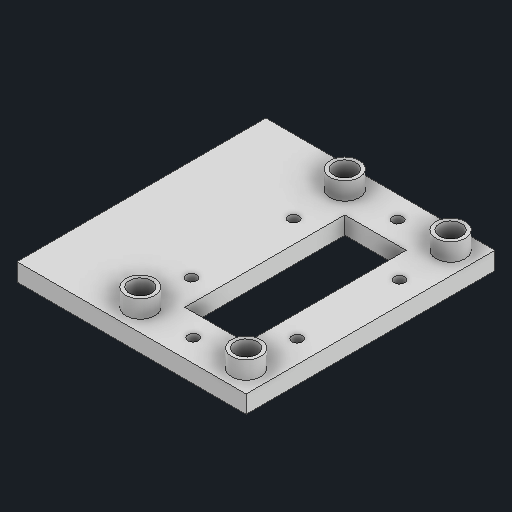
# Autodesk Inventor part: carriage_mount
Saved by Autodesk Inventor 2025 (Build 290162010, 162A)
## iProperties
Created: 2024-06-21
Part Number: carriage_mount
Material: Generic
Document SubType Name: Modeling
Designer: mihir
Density: 1 g/cm^3
Appearance: Default
Author: mihir
Autodesk Inventor part; units mm, degrees
ref_plane "YZ Plane" through (0, 0, 0) normal (1, 0, 0) x (0, 1, 0)
ref_plane "XZ Plane" through (0, 0, 0) normal (0, 1, 0) x (-1, 0, 0)
ref_plane "XY Plane" through (0, 0, 0) normal (0, 0, 1) x (1, 0, 0)
sketch "Sketch1" plane through (0, 0, 0) normal (0, 1, 0) x (-1, 0, 0)
  line L0 (0, 0) -> (65, 0)
  line L1 (65, 0) -> (65, -70.6)
  line L2 (65, -70.6) -> (0, -70.6)
  line L3 (0, -70.6) -> (0, 0)
  line L4 (30, -12.6) -> (12.6, -12.6)
  line L5 (12.6, -12.6) -> (12.6, -58)
  line L6 (12.6, -58) -> (30, -58)
  line L7 (30, -58) -> (30, -12.6)
  dimension "d0" = 70.6
  dimension "d1" = 65
  dimension "d2" = 45.4
  dimension "d3" = 17.4
  dimension "d4" = 12.6
  dimension "d5" = 12.6
  constraints: 16 end point, 4 parallel, 2 horizontal, 2 perpendicular
  measures "d0" distance of L2.end L0.start
  measures "d1" distance of L0.start L0.end
  measures "d2" distance of L4.end L5.end
  measures "d3" distance of L5.end L6.end
  measures "d4" distance between parallel lines of L2 L6
  measures "d5" distance between parallel lines of L3 L5
extrude "Extrusion1" add sketch "Sketch1" along normal blind 5
sketch "Sketch2" plane through (0, 5, 0) normal (0, 1, 0) x (1, 0, 0)
  line L0 (-12.6, 58) -> (-12.6, 12.6) construction
  line L1 (-12.6, 12.6) -> (0, 12.6) construction
  line L2 (0, 0) -> (0, 70.6) construction
  line L3 (-6.3, 6.3) -> (-6.3, 12.6) construction
  line L4 (-12.6, 12.6) -> (-30, 12.6) construction
  line L5 (-12.6, 12.6) -> (-12.6, 0) construction
  line L6 (-65, 0) -> (0, 0) construction
  line L7 (-6.3, 6.3) -> (-12.6, 6.3) construction
  line L8 (-6.3, 6.3) -> (-36.3, 6.3) construction
  line L9 (-36.3, 6.3) -> (-36.3, 64.3) construction
  line L10 (-36.3, 64.3) -> (-6.3, 64.3) construction
  line L11 (-6.3, 64.3) -> (-6.3, 6.3) construction
  line L12 (-6.3, 64.3) -> (-6.3, 70.6) construction
  line L13 (0, 70.6) -> (-65, 70.6) construction
  line L14 (-36.3, 35.3) -> (-30, 35.3) construction
  line L15 (-30, 12.6) -> (-30, 58) construction
  constraints: 20 end point, 4 horizontal, 4 midpoint, 4 vertical, 3 point on line, 2 equal length, 1 perpendicular
hole "Hole1" at (-36.3, 5, -6.3) at (-6.3, 5, -6.3) at (-36.3, 5, -64.3) at (-6.3, 5, -64.3) direction (0, -1, 0) diameter 6.3 depth 5
sketch "Sketch3" plane through (0, 5, 0) normal (0, 1, 0) x (1, 0, 0)
  circle A0 centre (-6.3, 6.3) radius 3.15 projected
  circle A1 centre (-6.3, 6.3) radius 4.15
  circle A2 centre (-36.3, 6.3) radius 3.15 projected
  circle A3 centre (-36.3, 6.3) radius 4.15
  circle A4 centre (-36.3, 64.3) radius 3.15 projected
  circle A5 centre (-36.3, 64.3) radius 4.15
  circle A6 centre (-6.3, 64.3) radius 3.15 projected
  circle A7 centre (-6.3, 64.3) radius 4.15
  point P0 (0, 0)
  dimension "d15" = 1
  constraints: 4 centre point, 4 coincident, 3 equal radius
  measures "d15" radial gap between concentric circles of A2 A3
extrude "Extrusion2" add sketch "Sketch3" along normal blind 5
sketch "Sketch4" plane through (0, 5, 0) normal (0, 1, 0) x (1, 0, 0)
  circle A0 centre (-36.3, 6.3) radius 4.15 construction
  circle A1 centre (-36.3, 64.3) radius 3.15 construction
  line L0 (-36.3, 6.3) -> (-36.3, 64.3) construction
  line L1 (-36.3, 64.3) -> (-6.3, 64.3) construction
  circle A2 centre (-6.3, 6.3) radius 3.15 construction
  line L2 (-36.3, 6.3) -> (-6.3, 6.3) construction
  circle A3 centre (-6.3, 64.3) radius 3.15 construction
  line L3 (-6.3, 6.3) -> (-6.3, 64.3) construction
  line L4 (-36.3, 35.3) -> (-6.3, 35.3) construction
  line L5 (-36.3, 20.8) -> (-6.3, 20.8) construction
  line L6 (-36.3, 49.8) -> (-6.3, 49.8) construction
  point P0 (0, 0)
  point P1 (-21.3, 64.3)
  point P2 (-21.3, 6.3)
  dimension "d18" = 14.5
  constraints: 14 end point, 4 midpoint, 4 point on line, 3 perpendicular, 2 horizontal, 1 vertical, 1 other
  measures "d18" distance between parallel lines of L2 L5
hole "Hole2" at (-36.3, 5, -20.8) at (-36.3, 5, -49.8) at (-6.3, 5, -20.8) at (-6.3, 5, -49.8) at (-21.3, 5, -64.3) at (-21.3, 5, -6.3) direction (0, -1, 0) diameter 3 depth 5
equation "\"d0\" = carriage_mount_width"
equation "\"d1\" = carriage_mount_length"
equation "\"d2\" = carriage_mount_cutout_length"
equation "\"d3\" = carriage_mount_cutout_width"
equation "\"d4\" = 0.5 * carriage_mount_width - 0.5 * carriage_mount_cutout_length"
equation "\"d5\" = 0.5 * carriage_mount_width - 0.5 * carriage_mount_cutout_length"
equation "\"d6\" = carriage_mount_thickness"
equation "\"d8\" = rod_diameter + rod_tolerance"
equation "\"d15\" = carriage_mount_wall_thickness"
equation "\"d16\" = carriage_mount_thickness"
equation "\"d18\" = 0.125 * carriage_mount_cutout_length + 0.125 * carriage_mount_width"
equation "\"d19\" = screw_diameter"
equation "\"carriage_mount_length\" = 65"
equation "\"carriage_mount_width\" = 70.6"
equation "\"carriage_mount_cutout_length\" = 45.4"
equation "\"carriage_mount_cutout_width\" = 17.4"
equation "\"screw_diameter\" = 3"
equation "\"rod_diameter\" = 6"
equation "\"rod_tolerance\" = 0.3"
equation "\"carriage_mount_wall_thickness\" = 1"
equation "\"carriage_mount_thickness\" = 5"
body "Solid1"
